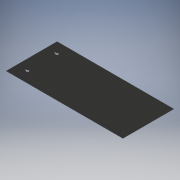
# Autodesk Inventor part: PRT1001-215 Base
Saved by Autodesk Inventor 2019 (Build 230136000, 136)
## iProperties
Created: 2019-07-02
Part Number: PRT1001-215 Base
Material: Generic
Document SubType Name: Modeling
Designer: james
Density: 1 g/cm^3
Appearance: Rubber - Black
Author: james
Autodesk Inventor part; units mm, degrees
ref_plane "YZ Plane" through (0, 0, 0) normal (1, 0, 0) x (0, 1, 0)
ref_plane "XZ Plane" through (0, 0, 0) normal (0, 1, 0) x (-1, 0, 0)
ref_plane "XY Plane" through (0, 0, 0) normal (0, 0, 1) x (1, 0, 0)
sketch "Sketch3" plane through (0, 0, 0) normal (0, 1, 0) x (-1, 0, 0)
  line L0 (447.8905, 299.355) -> (-108.1095, 299.355)
  line L1 (-108.1095, 299.355) -> (-108.1095, -348.645)
  line L2 (-108.1095, -348.645) -> (447.8905, -348.645)
  line L3 (447.8905, -348.645) -> (447.8905, 299.355)
  point P0 (0, 0)
  dimension "d19" = 648
  dimension "d20" = 556
  constraints: 8 end point, 2 parallel, 1 horizontal, 1 perpendicular
  measures "d19" distance of L0.end L1.end
  measures "d20" distance of L0.start L0.end
extrude "Extrusion2" add sketch "Sketch3" along normal blind 1
sketch "Sketch4" plane through (0, 1, 0) normal (0, 1, 0) x (1, 0, 0)
  line L0 (108.1095, 348.645) -> (-447.8905, 348.645) projected
  line L1 (108.1095, -299.355) -> (108.1095, 348.645) projected
  point P0 (84.1095, 324.645)
  point P1 (44.1095, 324.645)
  point P2 (44.1095, 132.645)
  point P3 (84.1095, 132.645)
  point P4 (34.1095, 322.645)
  point P5 (-3.8905, 322.645)
  point P6 (-3.8905, 132.645)
  point P7 (34.1095, 132.645)
  point P8 (-15.8905, 322.645)
  point P9 (-53.8905, 322.645)
  point P10 (-53.8905, 132.645)
  point P11 (-15.8905, 132.645)
  point P12 (-65.8905, 132.645)
  point P13 (-103.8905, 132.645)
  point P14 (-103.8905, 322.645)
  point P15 (-65.8905, 322.645)
  point P16 (-115.8905, 322.645)
  point P17 (-153.8905, 322.645)
  point P18 (-153.8905, 132.645)
  point P19 (-115.8905, 132.645)
  point P20 (-165.8905, 132.645)
  point P21 (-203.8905, 132.645)
  point P22 (-203.8905, 322.645)
  point P23 (-165.8905, 322.645)
  point P24 (-265.8905, 322.645)
  point P25 (-303.8905, 322.645)
  point P26 (-303.8905, 132.645)
  point P27 (-265.8905, 132.645)
  point P28 (-215.8905, 132.645)
  point P29 (-253.8905, 132.645)
  point P30 (-253.8905, 322.645)
  point P31 (-215.8905, 322.645)
  point P32 (-315.8905, 322.645)
  point P33 (-353.8905, 322.645)
  point P34 (-353.8905, 132.645)
  point P35 (-315.8905, 132.645)
  point P36 (-365.8905, 132.645)
  point P37 (-403.8905, 132.645)
  point P38 (-403.8905, 322.645)
  point P39 (-365.8905, 322.645)
  dimension "d23" = 24
  dimension "d24" = 24
  dimension "d34" = 0
  dimension "d35" = 0
  dimension "d36" = 0
  dimension "d37" = 0
  dimension "d38" = 192
  dimension "d39" = 40
  dimension "d60" = 0
  dimension "d61" = 0
  dimension "d62" = 0
  dimension "d63" = 0
  dimension "d64" = 190
  dimension "d65" = 38
  dimension "d91" = 0
  dimension "d92" = 0
  dimension "d93" = 0
  dimension "d94" = 0
  dimension "d95" = 190
  dimension "d96" = 38
  dimension "d113" = 0
  dimension "d114" = 0
  dimension "d115" = 0
  dimension "d116" = 0
  dimension "d117" = 190
  dimension "d118" = 38
  dimension "d153" = 0
  dimension "d154" = 0
  dimension "d155" = 0
  dimension "d156" = 0
  dimension "d157" = 190
  dimension "d158" = 38
  dimension "d175" = 0
  dimension "d176" = 0
  dimension "d177" = 0
  dimension "d178" = 0
  dimension "d179" = 190
  dimension "d180" = 38
  dimension "d199" = 0
  dimension "d200" = 0
  dimension "d201" = 0
  dimension "d202" = 0
  dimension "d203" = 190
  dimension "d204" = 38
  dimension "d221" = 0
  dimension "d222" = 0
  dimension "d223" = 0
  dimension "d224" = 0
  dimension "d225" = 190
  dimension "d226" = 38
  dimension "d275" = 0
  dimension "d276" = 0
  dimension "d277" = 0
  dimension "d278" = 0
  dimension "d279" = 190
  dimension "d280" = 38
  dimension "d297" = 0
  dimension "d298" = 0
  dimension "d299" = 0
  dimension "d300" = 0
  dimension "d301" = 190
  dimension "d302" = 38
  measures "d23" distance from line of L0 point (84.11, 324.645)
  measures "d24" distance from line of L1 point (84.11, 324.645)
  measures "d34" horizontal distance of point (84.11, 132.645) point (84.11, 324.645)
  measures "d35" horizontal distance of point (44.11, 324.645) point (44.11, 132.645)
  measures "d36" vertical distance of point (84.11, 324.645) point (44.11, 324.645)
  measures "d37" vertical distance of point (84.11, 132.645) point (44.11, 132.645)
  measures "d38" distance of point (84.11, 324.645) point (84.11, 132.645)
  measures "d39" distance of point (84.11, 324.645) point (44.11, 324.645)
  measures "d60" horizontal distance of point (34.11, 132.645) point (34.11, 322.645)
  measures "d61" horizontal distance of point (-3.89, 322.645) point (-3.89, 132.645)
  measures "d62" vertical distance of point (34.11, 322.645) point (-3.89, 322.645)
  measures "d63" vertical distance of point (34.11, 132.645) point (-3.89, 132.645)
  measures "d64" distance of point (34.11, 322.645) point (34.11, 132.645)
  measures "d65" distance of point (34.11, 322.645) point (-3.89, 322.645)
  measures "d91" horizontal distance of point (-15.89, 132.645) point (-15.89, 322.645)
  measures "d92" horizontal distance of point (-53.89, 322.645) point (-53.89, 132.645)
  measures "d93" vertical distance of point (-15.89, 322.645) point (-53.89, 322.645)
  measures "d94" vertical distance of point (-15.89, 132.645) point (-53.89, 132.645)
  measures "d95" distance of point (-15.89, 322.645) point (-15.89, 132.645)
  measures "d96" distance of point (-15.89, 322.645) point (-53.89, 322.645)
  measures "d113" horizontal distance of point (-65.89, 132.645) point (-65.89, 322.645)
  measures "d114" horizontal distance of point (-103.89, 322.645) point (-103.89, 132.645)
  measures "d115" vertical distance of point (-65.89, 322.645) point (-103.89, 322.645)
  measures "d116" vertical distance of point (-65.89, 132.645) point (-103.89, 132.645)
  measures "d117" distance of point (-65.89, 322.645) point (-65.89, 132.645)
  measures "d118" distance of point (-65.89, 322.645) point (-103.89, 322.645)
  measures "d153" horizontal distance of point (-115.89, 132.645) point (-115.89, 322.645)
  measures "d154" horizontal distance of point (-153.89, 322.645) point (-153.89, 132.645)
  measures "d155" vertical distance of point (-115.89, 322.645) point (-153.89, 322.645)
  measures "d156" vertical distance of point (-115.89, 132.645) point (-153.89, 132.645)
  measures "d157" distance of point (-115.89, 322.645) point (-115.89, 132.645)
  measures "d158" distance of point (-115.89, 322.645) point (-153.89, 322.645)
  measures "d175" horizontal distance of point (-165.89, 132.645) point (-165.89, 322.645)
  measures "d176" horizontal distance of point (-203.89, 322.645) point (-203.89, 132.645)
  measures "d177" vertical distance of point (-165.89, 322.645) point (-203.89, 322.645)
  measures "d178" vertical distance of point (-165.89, 132.645) point (-203.89, 132.645)
  measures "d179" distance of point (-165.89, 322.645) point (-165.89, 132.645)
  measures "d180" distance of point (-165.89, 322.645) point (-203.89, 322.645)
  measures "d199" horizontal distance of point (-215.89, 132.645) point (-215.89, 322.645)
  measures "d200" horizontal distance of point (-253.89, 322.645) point (-253.89, 132.645)
  measures "d201" vertical distance of point (-215.89, 322.645) point (-253.89, 322.645)
  measures "d202" vertical distance of point (-215.89, 132.645) point (-253.89, 132.645)
  measures "d203" distance of point (-215.89, 322.645) point (-215.89, 132.645)
  measures "d204" distance of point (-215.89, 322.645) point (-253.89, 322.645)
  measures "d221" horizontal distance of point (-265.89, 132.645) point (-265.89, 322.645)
  measures "d222" horizontal distance of point (-303.89, 322.645) point (-303.89, 132.645)
  measures "d223" vertical distance of point (-265.89, 322.645) point (-303.89, 322.645)
  measures "d224" vertical distance of point (-265.89, 132.645) point (-303.89, 132.645)
  measures "d225" distance of point (-265.89, 322.645) point (-265.89, 132.645)
  measures "d226" distance of point (-265.89, 322.645) point (-303.89, 322.645)
  measures "d275" horizontal distance of point (-315.89, 132.645) point (-315.89, 322.645)
  measures "d276" horizontal distance of point (-353.89, 322.645) point (-353.89, 132.645)
  measures "d277" vertical distance of point (-315.89, 322.645) point (-353.89, 322.645)
  measures "d278" vertical distance of point (-315.89, 132.645) point (-353.89, 132.645)
  measures "d279" distance of point (-315.89, 322.645) point (-315.89, 132.645)
  measures "d280" distance of point (-315.89, 322.645) point (-353.89, 322.645)
  measures "d297" horizontal distance of point (-365.89, 132.645) point (-365.89, 322.645)
  measures "d298" horizontal distance of point (-403.89, 322.645) point (-403.89, 132.645)
  measures "d299" vertical distance of point (-365.89, 322.645) point (-403.89, 322.645)
  measures "d300" vertical distance of point (-365.89, 132.645) point (-403.89, 132.645)
  measures "d301" distance of point (-365.89, 322.645) point (-365.89, 132.645)
  measures "d302" distance of point (-365.89, 322.645) point (-403.89, 322.645)
hole "Hole3" at (84.1095, 1, -324.645) at (44.1095, 1, -324.645) at (44.1095, 1, -132.645) at (84.1095, 1, -132.645) at (34.1095, 1, -132.645) at (-3.8905, 1, -132.645) at (-3.8905, 1, -322.645) at (34.1095, 1, -322.645) at (-65.8905, 1, -322.645) at (-103.8905, 1, -322.645) at (-103.8905, 1, -132.645) at (-65.8905, 1, -132.645) at (-15.8905, 1, -132.645) at (-53.8905, 1, -132.645) at (-53.8905, 1, -322.645) at (-15.8905, 1, -322.645) at (-215.8905, 1, -322.645) at (-253.8905, 1, -322.645) at (-253.8905, 1, -132.645) at (-215.8905, 1, -132.645) at (-265.8905, 1, -132.645) at (-303.8905, 1, -132.645) at (-303.8905, 1, -322.645) at (-265.8905, 1, -322.645) at (-165.8905, 1, -322.645) at (-203.8905, 1, -322.645) at (-203.8905, 1, -132.645) at (-165.8905, 1, -132.645) at (-115.8905, 1, -132.645) at (-153.8905, 1, -132.645) at (-153.8905, 1, -322.645) at (-115.8905, 1, -322.645) at (-365.8905, 1, -322.645) at (-403.8905, 1, -322.645) at (-403.8905, 1, -132.645) at (-365.8905, 1, -132.645) at (-315.8905, 1, -132.645) at (-353.8905, 1, -132.645) at (-353.8905, 1, -322.645) at (-315.8905, 1, -322.645) direction (0, -1, 0) diameter 3 depth 25.4 tip angle 118.188
sketch "Sketch6" plane through (0, 1, 0) normal (0, 1, 0) x (1, 0, 0)
  line L0 (-601.02, -516.5897) -> (252.7081, -516.5897)
  line L1 (252.7081, -516.5897) -> (252.7081, 106.645)
  line L2 (252.7081, 106.645) -> (-601.02, 106.645)
  line L3 (-601.02, 106.645) -> (-601.02, -516.5897)
  circle A0 centre (84.1095, 132.645) radius 1.5 projected
  point P0 (0, 0)
  dimension "d408" = 26
  constraints: 8 end point, 2 parallel, 1 horizontal, 1 perpendicular
  measures "d408" distance from line of L2 A0.centre
extrude "Extrusion3" cut sketch "Sketch6" against normal blind 25.4 contours L3 L2 L1 L0
sketch "Sketch7" plane through (0, 1, 0) normal (0, 1, 0) x (1, 0, 0)
  arc A0 (-402.5897, 154.27) -> (-402.5897, 160.62) centre (-397.0905, 157.445) ccw
  arc A1 (-402.5897, 294.67) -> (-402.5897, 301.02) centre (-397.0905, 297.845) ccw
  line L0 (108.1095, 348.645) -> (-447.8905, 348.645) projected
  line L1 (-447.8905, 348.645) -> (-447.8905, 106.645) projected
  line L2 (-447.8905, 106.645) -> (108.1095, 106.645) projected
  arc A2 (-407.2505, 160.62) -> (-407.2505, 154.27) centre (-407.2505, 157.445) ccw
  line L3 (-407.2505, 154.27) -> (-402.5897, 154.27)
  line L4 (-407.2505, 160.62) -> (-402.5897, 160.62)
  arc A3 (-407.2505, 301.02) -> (-407.2505, 294.67) centre (-407.2505, 297.845) ccw
  line L5 (-407.2505, 294.67) -> (-402.5897, 294.67)
  line L6 (-402.5897, 301.02) -> (-407.2505, 301.02)
  point P0 (0, 0)
  dimension "d411" = 12.7
  dimension "d412" = 50.8
  dimension "d413" = 50.8
  dimension "d414" = 50.8
  dimension "d415" = 50.8
  dimension "d416" = 12.7
  dimension "d417" = 6.35
  dimension "d418" = 0
  dimension "d419" = 10.16
  dimension "d420" = 6.35
  dimension "d421" = 0
  dimension "d422" = 10.16
  constraints: 8 end point, 8 point on circle, 4 centre point, 3 horizontal, 2 tangent, 1 parallel
  measures "d411" diameter of A1
  measures "d412" distance from line of A1.centre L0
  measures "d413" distance from line of A1.centre L1
  measures "d414" distance from line of L2 A0.centre
  measures "d415" distance from line of A0.centre L1
  measures "d416" diameter of A0
  measures "d417" diameter of A2
  measures "d418" vertical distance of A0.centre A2.centre
  measures "d419" distance of A0.centre A2.centre
  measures "d420" diameter of A3
  measures "d421" vertical distance of A1.centre A3.centre
  measures "d422" distance of A1.centre A3.centre
extrude "Extrusion4" cut sketch "Sketch7" against normal blind 25.4
equation "\"d19\" = BaseLength"
equation "\"d20\" = BaseWidth"
equation "\"d21\" = BoardHeight"
equation "\"d23\" = BaseBoardOffset + ScrewHoleOffset"
equation "\"d24\" = BaseBoardOffset + ScrewHoleOffset"
equation "\"d38\" = VertOffsetBetweenScrews"
equation "\"d39\" = HorizOffsetBetweenScrews"
equation "\"d64\" = d82"
equation "\"d65\" = d83"
equation "\"d95\" = d137"
equation "\"d96\" = d138"
equation "\"d117\" = d144"
equation "\"d118\" = d145"
equation "\"d157\" = d247"
equation "\"d158\" = d248"
equation "\"d179\" = d254"
equation "\"d180\" = d255"
equation "\"d203\" = d261"
equation "\"d204\" = d262"
equation "\"d225\" = d268"
equation "\"d226\" = d269"
equation "\"d279\" = d369"
equation "\"d280\" = d370"
equation "\"d301\" = d376"
equation "\"d302\" = d377"
equation "\"d401\" = ScrewSize"
equation "\"BoardWidth\" = 48"
equation "\"ScrewSize\" = 3"
equation "\"ScrewHoleOffset\" = 4"
equation "\"BoardGap\" = 4"
equation "\"BoardHeight\" = 1"
equation "\"BaseWidth\" = 556"
equation "\"HorizOffsetBetweenScrews\" = 40"
equation "\"VertOffsetBetweenScrews\" = 192"
equation "\"BaseBoardOffset\" = 20"
equation "\"BaseLength\" = 648"
equation "\"d47\" = 38"
equation "\"d55\" = 38"
equation "\"d82\" = 190"
equation "\"d83\" = 38"
equation "\"d85\" = 38"
equation "\"d87\" = 38"
equation "\"d88\" = 4"
equation "\"d137\" = 190"
equation "\"d138\" = 38"
equation "\"d140\" = 38"
equation "\"d142\" = 38"
equation "\"d143\" = 4"
equation "\"d144\" = 190"
equation "\"d145\" = 38"
equation "\"d147\" = 38"
equation "\"d149\" = 38"
equation "\"d150\" = 4"
equation "\"d247\" = 190"
equation "\"d248\" = 38"
equation "\"d250\" = 38"
equation "\"d252\" = 38"
equation "\"d253\" = 4"
equation "\"d254\" = 190"
equation "\"d255\" = 38"
equation "\"d257\" = 38"
equation "\"d259\" = 38"
equation "\"d260\" = 4"
equation "\"d261\" = 190"
equation "\"d262\" = 38"
equation "\"d264\" = 38"
equation "\"d266\" = 38"
equation "\"d267\" = 4"
equation "\"d268\" = 190"
equation "\"d269\" = 38"
equation "\"d271\" = 38"
equation "\"d273\" = 38"
equation "\"d274\" = 4"
equation "\"d369\" = 190"
equation "\"d370\" = 38"
equation "\"d372\" = 38"
equation "\"d374\" = 38"
equation "\"d375\" = 4"
equation "\"d376\" = 190"
equation "\"d377\" = 38"
equation "\"d379\" = 38"
equation "\"d381\" = 38"
equation "\"d382\" = 4"
equation "\"d384\" = 38"
equation "\"d386\" = 38"
equation "\"d388\" = 38"
equation "\"d389\" = 4"
equation "\"d391\" = 38"
equation "\"d393\" = 38"
equation "\"d395\" = 38"
equation "\"d396\" = 4"
body "Solid2"
